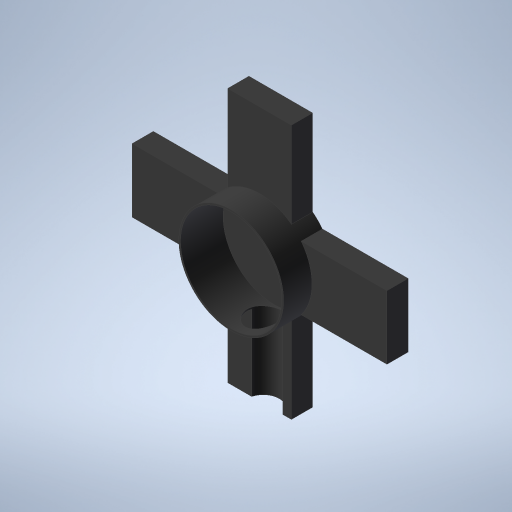
# Autodesk Inventor part: Part8
Saved by Autodesk Inventor 2024 (Build 280153000, 153)
## iProperties
Created: 2024-06-18
Part Number: Part8
Material: Generic
Document SubType Name: Sheet Metal
Designer: albah
Density: 1 g/cm^3
Sheet Metal Rule: Default_mm
Appearance: Default
Author: albah
Autodesk Inventor part; units mm, degrees
ref_plane "YZ Plane" through (0, 0, 0) normal (1, 0, 0) x (0, 1, 0)
ref_plane "XZ Plane" through (0, 0, 0) normal (0, 1, 0) x (-1, 0, 0)
ref_plane "XY Plane" through (0, 0, 0) normal (0, 0, 1) x (1, 0, 0)
sketch "Sketch1" plane through (0, 0, 0) normal (0, 0, 1) x (1, 0, 0)
  circle A0 centre (0, 0) radius 35.75
  circle A1 centre (0, 0) radius 37
  line L0 (-22.5, -90) -> (-22.5, 90)
  line L1 (-22.5, 90) -> (22.5, 90)
  line L2 (22.5, 90) -> (22.5, -90)
  line L3 (22.5, -90) -> (-22.5, -90)
  line L4 (-22.5, -90) -> (22.5, 90) construction
  line L5 (-22.5, 90) -> (22.5, -90) construction
  line L6 (-90, 22.5) -> (90, 22.5)
  line L7 (90, 22.5) -> (90, -22.5)
  line L8 (90, -22.5) -> (-90, -22.5)
  line L9 (-90, -22.5) -> (-90, 22.5)
  line L10 (-90, 22.5) -> (90, -22.5) construction
  line L11 (90, 22.5) -> (-90, -22.5) construction
  point P0 (22.5, -29.3726)
  point P1 (-22.5, -29.3726)
  point P2 (-29.3726, -22.5)
  point P3 (-29.3726, 22.5)
  point P4 (-22.5, 29.3726)
  point P5 (22.5, 29.3726)
  point P6 (29.3726, 22.5)
  point P7 (29.3726, -22.5)
  dimension "d0" = 71.5
  dimension "d1" = 74
  dimension "d2" = 180
  dimension "d3" = 45
  dimension "d4" = 180
  dimension "d5" = 45
  constraints: 24 end point, 5 parallel, 4 midpoint, 2 centre point, 2 coincident, 2 perpendicular, 1 vertical
  measures "d0" diameter of A0
  measures "d1" diameter of A1
  measures "d2" distance of L0.start L0.end
  measures "d3" distance of L0.end L1.end
  measures "d4" distance of L6.start L6.end
  measures "d5" distance of L6.end L7.end
extrude "Extrusion1" add sketch "Sketch1" along normal blind 5 contours A0 L8 L2 L6 | L6 L2 A0 | A0 L2 L8 | L2 L6 L0 A0 | L2 L8 L0 L6 | A0 L0 L8 L2 | L0 L6 A0 | L0 L8 A0 L6 | A0 L8 L0
extrude "Extrusion2" add sketch "Sketch1" along normal blind 30 contours A0 L6 A1 L8 | A0 L2 A1 L6 | L8 A1 L2 A0 | A0 L0 A1 L2 | L2 A1 L0 A0 | A0 L6 A1 L0 | L0 A1 L8 A0 | A0 L8 A1 L6
extrude "Extrusion3" add sketch "Sketch1" along normal blind 15 contours L6 L7 L8 A1 | A1 L0 L1 L2 | L2 L3 L0 A1 | A1 L8 L9 L6
sketch "Sketch2" plane through (-22.5, -90, 0) normal (0, -1, 0) x (1, 0, 0)
  point P0 (22.5, 0)
  point P1 (27.9129, 17.8091)
hole "Hole1" at (5.4129, -90, 17.8091) direction (0, 1, 0) diameter 22.606 depth 88.75 tip angle 118
move faces "Move1" translate (0, 0, 5) faces at (-36.0055, 0, 30)
equation "\"BendRadius\" = Thickness"
equation "\"BendReliefWidth\" = Thickness"
equation "\"BendReliefDepth\" = 0.5 * Thickness"
equation "\"CornerReliefSize\" = 4 * Thickness"
equation "\"MinimumRemnant\" = 2 * Thickness"
equation "\"TransitionRadius\" = BendRadius"
equation "\"JacobiRadiusSize\" = BendRadius"
equation "\"GapSize\" = Thickness"
equation "\"Thickness\" = 0.5"
body "Solid1"
